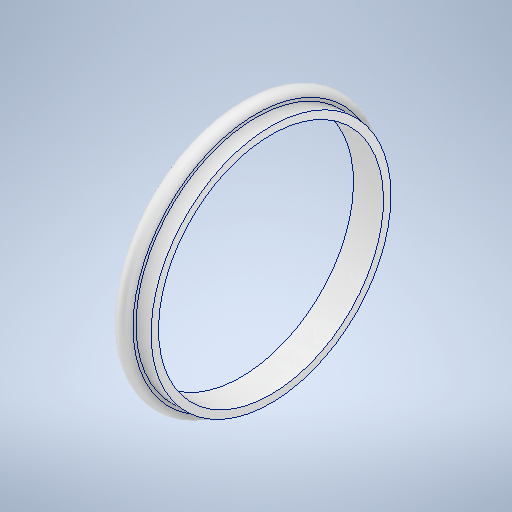
# Autodesk Inventor part: 1 part 29
Saved by Autodesk Inventor 2025.1 (Build 291241000, 241)
## iProperties
Created: 2024-08-01
Part Number: 1 part 29
Material: Aluminum 6061
Document SubType Name: Modeling
Designer: ffogue
Density: 2.7 g/cm^3
Appearance: Aluminum - Flat
Author: ffogue
Autodesk Inventor part; units mm, degrees
ref_plane "YZ Plane" through (0, 0, 0) normal (1, 0, 0) x (0, 1, 0)
ref_plane "XZ Plane" through (0, 0, 0) normal (0, 1, 0) x (-1, 0, 0)
ref_plane "XY Plane" through (0, 0, 0) normal (0, 0, 1) x (1, 0, 0)
sketch "Sketch1" plane through (0, 0, 0) normal (0, 0, 1) x (1, 0, 0)
  line L0 (0, 0) -> (5, 0)
  line L1 (5, 0) -> (5, 41)
  arc A0 (5, 41) -> (0, 41) centre (2.5, 41) ccw
  line L2 (0, 41) -> (0, 0)
  line L3 (5, 40) -> (10, 40)
  line L4 (10, 40) -> (10, 0)
  line L5 (10, 0) -> (5, 0)
  point P0 (2.5, 43.5)
  dimension "d0" = 5
  dimension "d5" = 87
  dimension "d6" = 80
  dimension "d7" = 5
  dimension "d8" = 2.5
  constraints: 12 end point, 5 perpendicular, 3 point on circle, 1 centre point, 1 horizontal, 1 point on line, 1 tangent
  measures "d0" distance between parallel lines of L1 L2
  measures "d5" diameter of point (2.5, 43.5) L0
  measures "d6" diameter of L3 L5
  measures "d7" distance of L3.start L3.end
  measures "d8" radius of A0
revolve "Revolution1" add sketch "Sketch1" angle 360 about axis through (0, 0, 0) along (1, 0, 0)
sketch "Sketch2" plane through (10, 0, 0) normal (1, 0, 0) x (0, 0, -1)
  circle A0 centre (0, 0) radius 40 projected
  constraints: 1 coincident
hole "Hole1" at (10, 0, 0) direction (-1, 0, 0) diameter 75 depth 10
body "Solid1"
